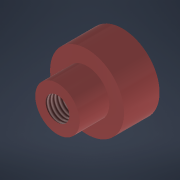
# Autodesk Inventor part: jack-pin
Saved by Autodesk Inventor 2021 (Build 250183000, 183)
## iProperties
Created: 2021-02-13
Part Number: jack-pin
Material: Generic
Document SubType Name: Modeling
Designer: vikki
Density: 1 g/cm^3
Appearance: Chestnut
Author: vikki
Autodesk Inventor part; units mm, degrees
ref_plane "YZ Plane" through (0, 0, 0) normal (1, 0, 0) x (0, 1, 0)
ref_plane "XZ Plane" through (0, 0, 0) normal (0, 1, 0) x (-1, 0, 0)
ref_plane "XY Plane" through (0, 0, 0) normal (0, 0, 1) x (1, 0, 0)
sketch "Sketch1" plane through (0, 0, 0) normal (0, 1, 0) x (-1, 0, 0)
  line L0 (0, 0) -> (0, -22)
  line L1 (4, 0) -> (7.5, 0)
  line L2 (7.5, 0) -> (7.5, -10)
  line L3 (7.5, -10) -> (12.5, -10)
  line L4 (12.5, -10) -> (12.5, -22)
  line L5 (12.5, -22) -> (9.5, -22)
  line L6 (9.5, -22) -> (9.5, -13)
  line L7 (9.5, -13) -> (4, -13)
  line L8 (4, -13) -> (4, 0)
  dimension "d0" = 3.5
  dimension "d1" = 3
  dimension "d2" = 12
  dimension "d3" = 10
  dimension "d4" = 3
  dimension "d5" = 25
  dimension "d6" = 15
  constraints: 18 end point, 7 perpendicular, 2 horizontal alignment, 1 horizontal, 1 vertical
  measures "d0" distance between parallel lines of L2 L8
  measures "d1" distance between parallel lines of L4 L6
  measures "d2" distance between parallel lines of L3 L5
  measures "d3" distance between parallel lines of L1 L3
  measures "d4" distance between parallel lines of L3 L7
  measures "d5" diameter of L4 L0
  measures "d6" diameter of L2 L0
revolve "Revolution1" add sketch "Sketch1" angle 360 about axis through (0, 0, 0) along (0, 0, -1)
thread "Thread1" size "M8x1.25" class "6H" standard "ANSI Metric M Profile" full length
body "Solid1"
